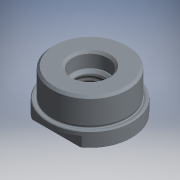
# Autodesk Inventor part: SLZ_63_Stopfen#
Saved by Autodesk Inventor 2017.3 (Build 213256000, 256)
## iProperties
Part Number: SLZ_63_Stopfen#
Material: Generic
Catalog Web Link: www.cadenas.de
Description: ProfilAbdeckstopfenSLZ63-Control-Tec
Vendor: ROSEKRIEGER
Document SubType Name: Modeling
Designer: partserver
Manufacturer: ROSEKRIEGER
Mass: 17.6586 g
Surface Area: 53.307 cm^2
Volume: 17.6586 cm^3
Density: 1 g/cm^3
Appearance: PSOLRGB-157-164-172
Category: PARTsolutions
Company: ROSEKRIEGER
Title: SLZ_63_Stopfen#
Author: Cadenas PARTsolutions
Comments: Control-Tec
PSOL_IDENT_0: {$CADENAS_DATA\23d-libs\rose_krieger\linearkomponenten\pool_lineartechnik\_hubsaeule_zyliinder\elekt
PSOL_IDENT_1: rozylinder\elekzyl_slz63\parts\slz63_plfl_stopfen.prj},188 {VTYP=3D},{NB=SLZ_63_Stopfen#},{LINA=SLZ_
PSOL_IDENT_2: 63_Stopfen#},{NN=ProfilAbdeckstopfenSLZ63},{DATE=02.12.2020 11:16:20},{GEOMDATE=08.03.2017 11:19:00}
PSOL_IDENT_3: ,{VERSION=},{LINEID=10},{WBVAR=},{WBNUMERIC=}  {NB=SLZ_63_Stopfen#},{LINA=SLZ_63_Stopfen#},{KT=DUMMY
PSOL_IDENT_4: },{IDNR=},{CODE=TQ3},{ARTIKEL=Elektrozylinder },{TYPE=SLZ 63 KG P PL},{BEST=SLZ_63_Stopfen},{VARIANT
PSOL_IDENT_5: E=PL},{SPINDEL=KG 25x10},{SPINDELCODE=3.000},{SCHUTZARTVIS=IP54},{SCHUTZART=1},{HUB1=0,[0:100]},{HIN
PSOL_IDENT_6: WEINBAUX=Hub + 288,5 mm},{DUMMYDURCH=10.000},{DUMMYLAENG=20.000},{HILFEHUB=105},{LAENDOPPROFIL=184.5
PSOL_IDENT_7: 00},{RF=1.000},{GRUNDKOE=288.500},{A=100},{B=80},{C=100},{D=125},{E=238},{F=40},{G=M16x1.5},{H=104},
PSOL_IDENT_8: {K=125},{L=105},{M=48},{N=56.5},{O=86},{P=18.5},{PPATH=sbl_lz70p_plfl.prj}
NB: SLZ_63_Stopfen#
NN: ProfilAbdeckstopfenSLZ63
NT: Control-Tec
NBSYN: $BEST.#
LINA: SLZ_63_Stopfen#
CATALOG: RK Rose+Krieger
ARTIKEL: Elektrozylinder
TYPE: SLZ 63 KG P PL
BEST: SLZ_63_Stopfen
VARIANTE: PL
SPINDEL: KG 25x10
SPINDELCODE: 3
SCHUTZARTVIS: IP54
SCHUTZART: 1
HUB1: 0,[0:100]
HINWEINBAUX: Hub + 288,5 mm
LAENDOPPROFIL: 184.5
RF: 1
GRUNDKOE: 288.5
A: 100
B: 80
C: 100
D: 125
E: 238
F: 40
G: M16x1.5
H: 104
K: 125
L: 105
M: 48
N: 56.5
O: 86
P: 18.5
SUPPLIER: ROSEKRIEGER
ARTICLENO: SLZ_63_Stopfen#
BOMINFO: SLZ_63_Stopfen#
CREATOR: CADENAS GmbH
Autodesk Inventor part; units mm, degrees
sketch "Sketch_3" plane through (0, 0, 0) normal (1, 0, 0) x (0, 0, -1)
  line L0 (13, 0) -> (-7, 0)
  line L1 (-7, 0) -> (-7, 19.7)
  line L2 (-7, 19.7) -> (-6.7, 20)
  line L3 (-6.7, 20) -> (-0.3, 20)
  line L4 (-0.3, 20) -> (0, 19.7)
  line L5 (0, 19.7) -> (0, 18.8198)
  line L6 (0, 18.8198) -> (-0.1759, 18.3366)
  arc A0 (-0.1759, 18.3366) -> (0.3035, 17.8134) centre (0.2, 18.1998) ccw
  line L7 (0.3035, 17.8134) -> (1, 18)
  line L8 (1, 18) -> (12, 18)
  line L9 (12, 18) -> (13, 17)
  line L10 (13, 17) -> (13, 0)
  line L11 (13, 0) -> (-7, 0)
  constraints: 24 end point, 2 point on circle, 1 centre point
revolve "Revolution1" add sketch "Sketch_3" angle 360 about axis through (0, 0, -13) along (0, 0, -1)
sketch "Sketch_1" plane through (0, 0, 0) normal (1, 0, 0) x (0, 0, -1)
  line L0 (13, 0) -> (-7, 0)
  line L1 (-7, 0) -> (-7, 8)
  line L2 (-7, 8) -> (-5.9175, 6.9175)
  line L3 (-5.9175, 6.9175) -> (4.9175, 6.9175)
  line L4 (4.9175, 6.9175) -> (6, 8)
  line L5 (6, 8) -> (6, 8.5)
  line L6 (6, 8.5) -> (12, 8.5)
  line L7 (12, 8.5) -> (13, 9.5)
  line L8 (13, 9.5) -> (13, 0)
  line L9 (13, 0) -> (-7, 0)
  constraints: 20 end point
revolve "Revolution2" cut sketch "Sketch_1" angle 360 about axis through (0, 0, -13) along (0, 0, -1)
thread "Thread1" size "M16x2" class "6H" standard "ISO Metric profile" full length
sketch "Sketch_6" plane through (0, 0, 0) normal (1, 0, 0) x (0, 0, -1)
  line L0 (-12, 25) -> (-12, -25)
  line L1 (-12, -25) -> (-2, -25)
  line L2 (-2, -25) -> (-2, -16)
  line L3 (-2, -16) -> (-7, -16)
  line L4 (-7, -16) -> (-7, 16)
  line L5 (-7, 16) -> (-2, 16)
  line L6 (-2, 16) -> (-2, 25)
  line L7 (-2, 25) -> (-12, 25)
  constraints: 16 end point
extrude "Extrusion1" cut sketch "Sketch_6" along normal mid plane 50
ref_plane "BP_POSHUB_ME_XY" through (0, 0, 7) normal (0, 0, 1) x (1, 0, 0)
ref_plane "BP_POSHUB_ME_YZ" through (0, 0, 7) normal (1, 0, 0) x (0, 1, 0)
ref_plane "BP_POSHUB_ME_ZX" through (0, 0, 7) normal (0, 1, 0) x (0, 0, 1)
ref_plane "DP401_XY" through (0, -16, 7) normal (1, 0, 0) x (0, 0, -1)
ref_plane "DP401_YZ" through (0, -16, 7) normal (0, 0, -1) x (0, 1, 0)
ref_plane "DP401_ZX" through (0, -16, 7) normal (0, 1, 0) x (1, 0, 0)
ref_plane "DPF1_XY" through (0, 20, 2) normal (1, 0, 0) x (0, 0, -1)
ref_plane "DPF1_YZ" through (0, 20, 2) normal (0, 0, -1) x (0, 1, 0)
ref_plane "DPF1_ZX" through (0, 20, 2) normal (0, 1, 0) x (1, 0, 0)
ref_plane "DPF2_XY" through (0, -20, 2) normal (1, 0, 0) x (0, 0, -1)
ref_plane "DPF2_YZ" through (0, -20, 2) normal (0, 0, -1) x (0, 1, 0)
ref_plane "DPF2_ZX" through (0, -20, 2) normal (0, 1, 0) x (1, 0, 0)
ref_plane "DPM2_XY" through (0, 16, 7) normal (1, 0, 0) x (0, 0, -1)
ref_plane "DPM2_YZ" through (0, 16, 7) normal (0, 0, -1) x (0, 1, 0)
ref_plane "DPM2_ZX" through (0, 16, 7) normal (0, 1, 0) x (1, 0, 0)
ref_plane "DPX2_XY" through (0, -16, 7) normal (1, 0, 0) x (0, 0, -1)
ref_plane "DPX2_YZ" through (0, -16, 7) normal (0, 0, -1) x (0, 1, 0)
ref_plane "DPX2_ZX" through (0, -16, 7) normal (0, 1, 0) x (1, 0, 0)
ref_plane "MUTTER_XY" through (0, 0, 7) normal (0, 0, -1) x (1, 0, 0)
ref_plane "MUTTER_YZ" through (0, 0, 7) normal (1, 0, 0) x (0, -1, 0)
ref_plane "MUTTER_ZX" through (0, 0, 7) normal (0, -1, 0) x (0, 0, -1)
ref_plane "SCHRAUBE_XY" through (0, 0, -13) normal (0, 0, 1) x (1, 0, 0)
ref_plane "SCHRAUBE_YZ" through (0, 0, -13) normal (1, 0, 0) x (0, 1, 0)
ref_plane "SCHRAUBE_ZX" through (0, 0, -13) normal (0, 1, 0) x (0, 0, 1)
ref_plane "SCHUBSTANGE_XY" through (0, 0, 0) normal (0, 0, 1) x (1, 0, 0)
ref_plane "SCHUBSTANGE_YZ" through (0, 0, 0) normal (1, 0, 0) x (0, 1, 0)
ref_plane "SCHUBSTANGE_ZX" through (0, 0, 0) normal (0, 1, 0) x (0, 0, 1)
ref_plane "STOPFEN_XY" through (0, 0, 7) normal (0, 0, -1) x (1, 0, 0)
ref_plane "STOPFEN_YZ" through (0, 0, 7) normal (1, 0, 0) x (0, -1, 0)
ref_plane "STOPFEN_ZX" through (0, 0, 7) normal (0, -1, 0) x (0, 0, -1)
body "Solid1"
